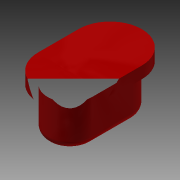
# Autodesk Inventor part: LCDButton
Saved by Autodesk Inventor 2015 SP1 (Build 190203100, 203)
## iProperties
Created: 2015-04-17
Part Number: LCDButton
Material: ABS Plastic
Document SubType Name: Modeling
Designer: Jack
Density: 1.06 g/cm^3
Appearance: Smooth - Red
Author: Jack
Autodesk Inventor part; units mm, degrees
ref_plane "YZ Plane" through (0, 0, 0) normal (1, 0, 0) x (0, 1, 0)
ref_plane "XZ Plane" through (0, 0, 0) normal (0, 1, 0) x (-1, 0, 0)
ref_plane "XY Plane" through (0, 0, 0) normal (0, 0, 1) x (1, 0, 0)
sketch "Sketch1" plane through (0, 0, 0) normal (0, 0, 1) x (1, 0, 0)
  line L0 (0, -2.55) -> (0, 2.55) construction
  line L1 (4, -2.55) -> (4, 2.55)
  line L2 (-4, 2.55) -> (-4, -2.55)
  arc A0 (-4, -2.55) -> (4, -2.55) centre (0, -2.55) ccw
  arc A1 (4, 2.55) -> (-4, 2.55) centre (0, 2.55) ccw
  point P0 (0, 0)
  dimension "d0" = 2.55
  dimension "d1" = 8
  constraints: 8 end point, 4 point on circle, 4 tangent, 2 centre point, 1 midpoint, 1 parallel, 1 vertical
  measures "d0" distance of point (0, 0) L0.end
  measures "d1" diameter of A1
extrude "Extrusion1" add sketch "Sketch1" along normal blind 1.5
sketch "Sketch2" plane through (0, 0, 0) normal (0, 0, -1) x (-1, 0, 0)
  line L0 (-4, -2.55) -> (-4, 2.55) projected
  arc A0 (-4, -2.55) -> (4, -2.55) centre (0, -2.55) ccw projected
  line L1 (4, 2.55) -> (4, -2.55) projected
  arc A1 (4, 2.55) -> (-4, 2.55) centre (0, 2.55) ccw projected
  line L2 (-2.8, 2.55) -> (-2.8, -2.55)
  arc A2 (-2.8, -2.55) -> (2.8, -2.55) centre (0, -2.55) ccw
  line L3 (2.8, -2.55) -> (2.8, 2.55)
  arc A3 (2.8, 2.55) -> (-2.8, 2.55) centre (0, 2.55) ccw
  point P0 (0, 0)
  dimension "d4" = 1.2
  constraints: 4 end point, 4 point on circle, 2 centre point, 3 other
  measures "d4" radial gap between concentric circles of A1 A3
extrude "Extrusion2" add sketch "Sketch2" along normal blind 5.3 contours A3 L3 A2 L2
fillet "Fillet1" radius 1 4 edges at (2.8, 0, -5.3) (0, -5.35, -5.3) (-2.8, 0, -5.3) (0, 5.35, -5.3)
body "Solid1"
